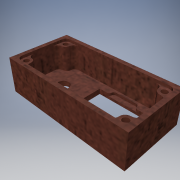
# Autodesk Inventor part: Display Case
Saved by Autodesk Inventor 2019 (Build 230136000, 136)
## iProperties
Created: 2019-03-05
Part Number: Display Case
Material: Wood (Walnut)
Document SubType Name: Modeling
Designer: Jackson Smith
Density: 0.55 g/cm^3
Appearance: Walnut - Stained Light No Gloss
Author: Jackson Smith
Autodesk Inventor part; units mm, degrees
ref_plane "YZ Plane" through (0, 0, 0) normal (1, 0, 0) x (0, 1, 0)
ref_plane "XZ Plane" through (0, 0, 0) normal (0, 1, 0) x (-1, 0, 0)
ref_plane "XY Plane" through (0, 0, 0) normal (0, 0, 1) x (1, 0, 0)
sketch "Sketch1" plane through (0, 0, 0) normal (0, 1, 0) x (-1, 0, 0)
  line L0 (35, -17.5) -> (-35, -17.5)
  line L1 (-35, -17.5) -> (-35, 17.5)
  line L2 (-35, 17.5) -> (35, 17.5)
  line L3 (35, 17.5) -> (35, -17.5)
  line L4 (35, -17.5) -> (-35, 17.5) construction
  line L5 (-35, -17.5) -> (35, 17.5) construction
  point P0 (0, 0)
  dimension "d0" = 70
  dimension "d1" = 35
  constraints: 12 end point, 2 midpoint, 2 parallel, 1 horizontal, 1 perpendicular
  measures "d0" distance of L0.start L0.end
  measures "d1" distance of L2.end L0.start
extrude "Extrusion1" add sketch "Sketch1" along normal blind 19.05
sketch "Sketch2" plane through (0, 19.05, 0) normal (0, 1, 0) x (1, 0, 0)
  line L0 (32.5, -15) -> (-32.5, -15)
  line L1 (-32.5, -15) -> (-32.5, 15)
  line L2 (-32.5, 15) -> (32.5, 15)
  line L3 (32.5, 15) -> (32.5, -15)
  line L4 (32.5, -15) -> (-32.5, 15) construction
  line L5 (-32.5, -15) -> (32.5, 15) construction
  point P0 (0, 0)
  dimension "d4" = 65
  dimension "d5" = 30
  constraints: 12 end point, 2 midpoint, 2 parallel, 1 horizontal, 1 perpendicular
  measures "d4" distance of L1.end L2.end
  measures "d5" distance of L0.end L1.end
extrude "Extrusion2" cut sketch "Sketch2" against normal blind 1.5875
fillet "Fillet1" radius 3 4 edges at (-32.5, 18.2563, -15) (-32.5, 18.2563, 15) (32.5, 18.2563, -15) (32.5, 18.2563, 15)
sketch "Sketch3" plane through (0, 17.4625, 0) normal (0, 1, 0) x (1, 0, 0)
  arc A0 (-29.5, 15) -> (-32.5, 12) centre (-29.5, 12) ccw projected
  arc A1 (-32.5, -12) -> (-29.5, -15) centre (-29.5, -12) ccw projected
  arc A2 (29.5, -15) -> (32.5, -12) centre (29.5, -12) ccw projected
  arc A3 (32.5, 12) -> (29.5, 15) centre (29.5, 12) ccw projected
  point P0 (0, 0)
  constraints: 4 coincident
hole "Hole1" at (-29.5, 17.4625, -12) at (-29.5, 17.4625, 12) at (29.5, 17.4625, 12) at (29.5, 17.4625, -12) direction (0, -1, 0) diameter 3.175 depth 15.875
sketch "Sketch4" plane through (0, 17.4625, 0) normal (0, 1, 0) x (1, 0, 0)
  circle A0 centre (-29.5, 12) radius 1.5875 construction
  circle A1 centre (-29.5, 12) radius 3
  circle A2 centre (-29.5, -12) radius 1.5875 construction
  circle A3 centre (-29.5, -12) radius 3
  circle A4 centre (29.5, -12) radius 1.5875 construction
  arc A5 (29.5, -15) -> (32.5, -12) centre (29.5, -12) ccw projected
  circle A6 centre (29.5, -12) radius 3
  circle A7 centre (29.5, 12) radius 1.5875 construction
  circle A8 centre (29.5, 12) radius 3
  arc A9 (-29.5, 15) -> (-32.5, 12) centre (-29.5, 12) ccw projected
  arc A10 (-32.5, -12) -> (-29.5, -15) centre (-29.5, -12) ccw projected
  arc A11 (32.5, 12) -> (29.5, 15) centre (29.5, 12) ccw projected
  line L0 (-29.5, 15) -> (29.5, 15) projected
  line L1 (-29.5, 15) -> (29.5, 15)
  line L2 (-35, 17.5) -> (35, 17.5) projected
  line L3 (-32.5, -12) -> (-32.5, 12) projected
  line L4 (-32.5, 12) -> (-32.5, -12)
  arc A12 (-32.5, -12) -> (-29.5, -15) centre (-29.5, -12) ccw projected
  line L5 (-29.5, -15) -> (29.5, -15)
  line L6 (32.5, 12) -> (32.5, -12) projected
  line L7 (32.5, 12) -> (32.5, -12)
  point P0 (0, 0)
  point P1 (-29.5, -9)
  point P2 (-26.5, -12)
  point P3 (-29.5, 9)
  point P4 (-26.5, 12)
  point P5 (26.5, 12)
  point P6 (29.5, 9)
  point P7 (26.5, -12)
  point P8 (29.5, -9)
  constraints: 9 point on circle, 8 end point, 6 tangent, 4 centre point, 4 coincident, 3 concentric, 2 collinear, 2 horizontal alignment, 2 vertical alignment, 1 horizontal, 1 parallel
extrude "Extrusion3" cut sketch "Sketch4" against normal blind 14.2875 contours A1 L0 A8 L6 A6 L5 A3 L3
fillet "Fillet3" radius 3 8 edges at (-32.5, 10.3188, -12) (-29.5, 10.3188, -15) (-32.5, 10.3188, 12) (-29.5, 10.3188, 15) (29.5, 10.3188, 15) (32.5, 10.3188, 12) (29.5, 10.3188, -15) (32.5, 10.3188, -12)
sketch "Sketch6" plane through (0, 3.175, 0) normal (0, 1, 0) x (1, 0, 0)
  line L0 (-3.75, 10.5) -> (23.75, 10.5)
  line L1 (23.75, 10.5) -> (23.75, -10.5)
  line L2 (23.75, -10.5) -> (-3.75, -10.5)
  line L3 (-3.75, -10.5) -> (-3.75, 10.5)
  line L4 (-3.75, 10.5) -> (23.75, -10.5) construction
  line L5 (23.75, 10.5) -> (-3.75, -10.5) construction
  line L6 (-3.5, 14) -> (23.5, 14) construction
  line L7 (23.5, 14) -> (23.5, -14) construction
  line L8 (23.5, -14) -> (-3.5, -14) construction
  line L9 (-3.5, -14) -> (-3.5, 14) construction
  line L10 (-3.5, 14) -> (23.5, -14) construction
  line L11 (23.5, 14) -> (-3.5, -14) construction
  point P0 (0, 0)
  point P1 (10, 0)
  point P2 (10, 0)
  point P3 (10, 0)
  dimension "d22" = 27.5
  dimension "d23" = 21
  dimension "d24" = 27
  dimension "d25" = 28
  dimension "d26" = 10
  constraints: 24 end point, 6 midpoint, 4 parallel, 2 horizontal, 2 perpendicular, 1 horizontal alignment
  measures "d22" distance of L1.end L2.end
  measures "d23" distance of L0.end L1.end
  measures "d24" distance of L7.end L8.end
  measures "d25" distance of L6.end L7.end
  measures "d26" distance of point (10, 0) point (0, 0)
extrude "Extrusion4" cut sketch "Sketch6" against normal through all
sketch "Sketch7" plane through (0, 3.175, 0) normal (0, 1, 0) x (1, 0, 0)
  line L0 (-3.75, -10.5) -> (-3.75, 10.5) projected
  point P0 (0, 0)
  point P1 (-18.75, 0)
  dimension "d37" = 15
  constraints: 1 horizontal alignment
  measures "d37" distance from line of point (-18.75, 0) L0
hole "Hole2" at (-18.75, 3.175, 0) direction (0, -1, 0) diameter 7.5 end through all
sketch "Sketch8" plane through (0, 3.175, 0) normal (0, 1, 0) x (1, 0, 0)
  line L0 (17.5, 13.5) -> (2.5, 13.5)
  line L1 (2.5, 13.5) -> (2.5, 10.5)
  line L2 (2.5, 10.5) -> (17.5, 10.5)
  line L3 (17.5, 10.5) -> (17.5, 13.5)
  line L4 (-3.75, 10.5) -> (23.75, 10.5) projected
  point P0 (0, 0)
  point P1 (10, 13.5)
  point P2 (10, 10.5)
  point P3 (10, 10.5)
  dimension "d38" = 3
  dimension "d39" = 15
  constraints: 8 end point, 4 midpoint, 2 parallel, 1 horizontal, 1 perpendicular, 1 vertical alignment
  measures "d38" distance of L1.end L0.end
  measures "d39" distance of L1.end L2.end
extrude "Extrusion5" cut sketch "Sketch8" against normal blind 1.5875
fillet "Fillet5" radius 1.5875 4 edges at (2.5, 2.3812, -13.5) (2.5, 2.3812, -10.5) (17.5, 2.3812, -13.5) (17.5, 2.3812, -10.5)
body "Solid1"
